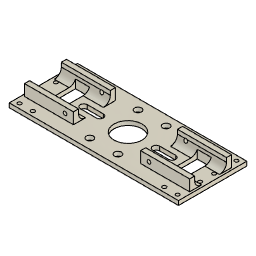
电路板支撑架 v2 (Autodesk Fusion 360 design; units mm, degrees)
Autodesk Fusion 360 part; units mm, degrees
sketch "草图1" plane through (0, 0, 0) normal (0, 0, 1) x (1, 0, 0)
  line L0 (-76.346, 23.9106) -> (50.654, 23.9106)
  line L1 (50.654, 23.9106) -> (50.654, -24.8894)
  line L2 (50.654, -24.8894) -> (-76.346, -24.8894)
  line L3 (-76.346, -24.8894) -> (-76.346, 23.9106)
  dimension "d1" = 127
  dimension "d2" = 48.8
  constraint horizontal L0
  constraint vertical L1
  constraint horizontal L2
  constraint vertical L3
  measures "d1" distance of L0.start L0.end
  measures "d2" distance of L0.start L2.end
extrude "拉伸1" add sketch "草图1" along normal blind 3
sketch "草图2" plane through (0, 0, 3) normal (0, 0, 1) x (-1, 0, 0)
  line L0 (76.346, 24.8894) -> (-50.654, 24.8894)
  line L1 (-50.654, 24.8894) -> (-50.654, -23.9106)
  line L2 (-50.654, -23.9106) -> (76.346, -23.9106)
  line L3 (76.346, -23.9106) -> (76.346, 24.8894)
  line L4 (12.846, -23.9106) -> (12.846, 24.8894) construction
  line L5 (76.346, 0.4894) -> (12.846, 0.4894) construction
  line L6 (12.846, 0.4894) -> (12.846, -12.4106)
  line L7 (-50.654, -10.9106) -> (76.346, -10.9106)
  line L8 (76.346, -10.9106) -> (76.346, -13.9106)
  line L9 (76.346, -13.9106) -> (-50.654, -13.9106)
  line L10 (-50.654, -13.9106) -> (-50.654, -10.9106)
  line L11 (-50.654, -10.9106) -> (76.346, -13.9106) construction
  line L12 (76.346, -10.9106) -> (-50.654, -13.9106) construction
  line L13 (12.846, 0.4894) -> (12.846, 13.3894)
  line L14 (-50.654, 14.8894) -> (76.346, 14.8894)
  line L15 (76.346, 14.8894) -> (76.346, 11.8894)
  line L16 (76.346, 11.8894) -> (-50.654, 11.8894)
  line L17 (-50.654, 11.8894) -> (-50.654, 14.8894)
  line L18 (-50.654, 14.8894) -> (76.346, 11.8894) construction
  line L19 (76.346, 14.8894) -> (-50.654, 11.8894) construction
  point P0 (12.846, -12.4106)
  point P1 (12.846, 13.3894)
  dimension "d5" = 12.9
  dimension "d6" = 3
  dimension "d7" = 3
  constraint midpoint L2 L4.start
  constraint midpoint L0 L4.end
  constraint midpoint L3 L5.start
  constraint midpoint L4 L5.end
  constraint perpendicular L5 L6
  constraint horizontal L7
  constraint perpendicular L7 L8
  constraint parallel L7 L9
  constraint parallel L8 L10
  constraint coincident L11 P0
  constraint coincident L12 P0
  constraint coincident P0 L6.end
  constraint symmetric L6.start L5 L13.start
  constraint symmetric L5 P0 P1
  constraint horizontal L14
  constraint perpendicular L14 L15
  constraint parallel L14 L16
  constraint parallel L15 L17
  constraint coincident L18 P1
  constraint coincident L19 P1
  constraint coincident P1 L13.end
  measures "d5" distance of L5.end P0
  measures "d6" distance of L7.end L8.end
  measures "d7" distance of L14.end L15.end
extrude "拉伸2" add sketch "草图2" along normal blind 8 contours L1 L3 L14 L15 L16 L17 | L1 L3 L7 L8 L9 L10
sketch "草图3" plane through (0, -14.8894, 0) normal (0, -1, 0) x (1, 0, 0)
  line L0 (-76.346, 3) -> (50.654, 3)
  line L1 (50.654, 3) -> (50.654, 11)
  line L2 (50.654, 11) -> (-76.346, 11)
  line L3 (-76.346, 11) -> (-76.346, 3)
  line L4 (-12.846, 11) -> (-12.846, 7)
  line L5 (-12.846, 7) -> (17.154, 7) construction
  circle A0 centre (17.154, 7) radius 1.3
  circle A1 centre (-42.846, 7) radius 1.3
  dimension "d13" = 4
  dimension "d14" = 30
  dimension "d15" = 2.6
  constraint midpoint L2 L4.start
  constraint perpendicular L2 L4
  constraint perpendicular L4 L5
  constraint coincident L5.end A0.centre
  constraint symmetric L4 A0 A1
  measures "d13" distance of L4.start L4.end
  measures "d14" distance of L4.end L5.end
  measures "d15" diameter of A0
extrude "拉伸3" cut sketch "草图3" against normal blind 28.8 contours A0 | A1
sketch "草图4" plane through (0, 13.9106, 0) normal (0, 1, 0) x (-1, 0, 0)
  circle A0 centre (-17.154, 7) radius 1.3
  circle A1 centre (42.846, 7) radius 1.3
  line L0 (-50.654, 3) -> (76.346, 3)
  line L1 (76.346, 3) -> (76.346, 11)
  line L2 (76.346, 11) -> (-50.654, 11)
  line L3 (-50.654, 11) -> (-50.654, 3)
  line L4 (12.846, 3) -> (12.846, 26.5) construction
  circle A2 centre (12.846, 26.5) radius 21
  dimension "d20" = 23.5
  dimension "d21" = 42
  constraint midpoint L0 L4.start
  constraint perpendicular L2 L4
  constraint coincident L4.end A2.centre
  measures "d20" distance of L4.start L4.end
  measures "d21" diameter of A2
sketch "草图5" plane through (0, 0, 0) normal (0, 0, -1) x (1, 0, 0)
  line L0 (50.654, 24.8894) -> (-76.346, 24.8894)
  line L1 (-76.346, 24.8894) -> (-76.346, -23.9106)
  line L2 (-76.346, -23.9106) -> (50.654, -23.9106)
  line L3 (50.654, -23.9106) -> (50.654, 24.8894)
  line L4 (-12.846, -23.9106) -> (-12.846, -3)
  line L5 (50.654, 0.4894) -> (30.654, 0.4894) construction
  line L6 (25.654, 11.4894) -> (35.654, 11.4894)
  line L7 (35.654, 11.4894) -> (35.654, -10.5106)
  line L8 (35.654, -10.5106) -> (25.654, -10.5106)
  line L9 (25.654, -10.5106) -> (25.654, 11.4894)
  line L10 (25.654, 11.4894) -> (35.654, -10.5106) construction
  line L11 (35.654, 11.4894) -> (25.654, -10.5106) construction
  line L12 (-51.346, -10.5106) -> (-51.346, 11.4894)
  line L13 (-61.346, -10.5106) -> (-51.346, -10.5106)
  line L14 (-61.346, 11.4894) -> (-61.346, -10.5106)
  line L15 (-51.346, 11.4894) -> (-61.346, 11.4894)
  circle A0 centre (-12.846, 0.4894) radius 10
  line L16 (30.654, 0.4894) -> (-51.346, 0.4894)
  line L17 (-12.846, -3) -> (-12.846, 0.4894)
  line L18 (-76.346, 24.8894) -> (-71.846, 24.8894)
  line L19 (-71.846, 24.8894) -> (-71.846, -23.9106)
  line L20 (-71.846, -23.9106) -> (-76.346, -23.9106)
  line L21 (-76.346, -23.9106) -> (-76.346, 24.8894)
  line L22 (46.154, 24.8894) -> (46.154, -23.9106)
  line L23 (50.654, -23.9106) -> (50.654, 24.8894)
  line L24 (50.654, 24.8894) -> (46.154, 24.8894)
  line L25 (46.154, -23.9106) -> (50.654, -23.9106)
  point P0 (30.654, 0.4894)
  dimension "d24" = 20
  dimension "d25" = 10
  dimension "d26" = 22
  dimension "d29" = 20
  dimension "d54" = 4.5
  dimension "d55" = 48.8
  constraint midpoint L2 L4.start
  constraint perpendicular L2 L4
  constraint midpoint L3 L5.start
  constraint perpendicular L3 L5
  constraint horizontal L6
  constraint perpendicular L6 L7
  constraint parallel L6 L8
  constraint parallel L7 L9
  constraint coincident L10 P0
  constraint coincident L11 P0
  constraint coincident P0 L5.end
  constraint symmetric L4 L6.start L12.end
  constraint symmetric L4 L6.end L14.start
  constraint symmetric L4 L7.end L13.start
  constraint symmetric L4 L8.end L12.start
  constraint midpoint L12 L16.end
  constraint coincident A0.centre L16
  constraint coincident L16 A0.centre
  constraint perpendicular L16 L17
  constraint coincident A0.centre L17.end
  constraint horizontal L18
  constraint vertical L19
  constraint horizontal L20
  constraint vertical L21
  constraint coincident L0.end L1.start
  constraint symmetric L17 L0.end L0.start
  constraint symmetric L17 L18.end L22.start
  constraint symmetric L17 L19.end L22.end
  constraint symmetric L17 L1.end L2.end
  measures "d24" distance of L5.start P0
  measures "d25" distance of L7.end L8.end
  measures "d26" distance of L6.end L7.end
  measures "d29" diameter of A0
  measures "d54" distance of L0.end L18.end
  measures "d55" distance of L0.end L1.end
extrude "拉伸5" cut sketch "草图5" against normal blind 3 contours L6 L7 L8 L9 | L12 L13 L14 L15
extrude "拉伸6" cut sketch "草图5" against normal blind 3 contours L4 A0 L16 L17 | L4 A0 L16 L17 | A0 L16
fillet "圆角2" radius 5 2 edges at (-12.846, 10.9106, 3) (-12.846, -11.8894, 3)
sketch "草图6" plane through (0, -14.8894, 0) normal (0, -1, 0) x (1, 0, 0)
  circle A0 centre (17.154, 7) radius 1.3
  circle A1 centre (-42.846, 7) radius 1.3
  line L0 (-76.346, 3) -> (50.654, 3)
  line L1 (50.654, 3) -> (50.654, 11)
  line L2 (50.654, 11) -> (-76.346, 11)
  line L3 (-76.346, 11) -> (-76.346, 3)
  line L4 (17.154, 7) -> (-12.846, 7)
  line L5 (11.154, 11) -> (-36.846, 11)
  line L6 (-36.846, 11) -> (-36.846, 3)
  line L7 (-36.846, 3) -> (11.154, 3)
  line L8 (11.154, 3) -> (11.154, 11)
  line L9 (11.154, 11) -> (-36.846, 3) construction
  line L10 (-36.846, 11) -> (11.154, 3) construction
  point P0 (-12.846, 7)
  dimension "d34" = 30
  dimension "d35" = 48
  constraint coincident A0.centre L4.start
  constraint parallel L0 L4
  constraint horizontal L5
  constraint perpendicular L5 L6
  constraint parallel L5 L7
  constraint parallel L6 L8
  constraint coincident L9 P0
  constraint coincident L10 P0
  constraint coincident L2 L5.start
  constraint coincident P0 L4.end
  measures "d34" distance of A0.centre P0
  measures "d35" distance of L6.end L7.end
extrude "拉伸7" cut sketch "草图6" against normal blind 28.8 contours L0 L2 L5 L6 L7 L8
sketch "草图7" plane through (0, 0, 0) normal (0, 0, -1) x (1, 0, 0)
  circle A0 centre (-12.846, 0.4894) radius 10
  line L0 (-61.346, -10.5106) -> (-61.346, 11.4894)
  line L1 (-61.346, 11.4894) -> (-51.346, 11.4894)
  line L2 (-51.346, 11.4894) -> (-51.346, -10.5106)
  line L3 (-51.346, -10.5106) -> (-61.346, -10.5106)
  line L4 (35.654, 11.4894) -> (35.654, -10.5106)
  line L5 (35.654, -10.5106) -> (25.654, -10.5106)
  line L6 (25.654, -10.5106) -> (25.654, 11.4894)
  line L7 (25.654, 11.4894) -> (35.654, 11.4894)
  line L8 (50.654, 24.8894) -> (-76.346, 24.8894)
  line L9 (-76.346, 24.8894) -> (-76.346, -23.9106)
  line L10 (-76.346, -23.9106) -> (50.654, -23.9106)
  line L11 (50.654, -23.9106) -> (50.654, 24.8894)
  line L12 (34.154, -20.5106) -> (-59.846, -20.5106) construction
  line L13 (-59.846, -20.5106) -> (-59.846, 21.4894) construction
  line L14 (-59.846, 21.4894) -> (34.154, 21.4894) construction
  line L15 (34.154, 21.4894) -> (34.154, -20.5106) construction
  line L16 (34.154, -20.5106) -> (-59.846, 21.4894) construction
  line L17 (-59.846, -20.5106) -> (34.154, 21.4894) construction
  circle A1 centre (-59.846, 21.4894) radius 1.4
  circle A2 centre (34.154, 21.4894) radius 1.4
  circle A3 centre (34.154, -20.5106) radius 1.4
  circle A4 centre (-59.846, -20.5106) radius 1.4
  point P0 (-12.846, 0.4894)
  dimension "d38" = 94
  dimension "d39" = 42
  dimension "d40" = 2.8
  dimension "d41" = 2.8
  dimension "d42" = 2.8
  dimension "d43" = 2.8
  constraint horizontal L12
  constraint perpendicular L12 L13
  constraint parallel L12 L14
  constraint parallel L13 L15
  constraint coincident L16 P0
  constraint coincident L17 P0
  constraint coincident P0 A0.centre
  constraint coincident L13.end L14.start
  constraint coincident L14.end L15.start
  constraint coincident L12.start L15.end
  constraint coincident L12.end L13.start
  measures "d38" distance of L13.end L14.end
  measures "d39" distance of L12.end L13.end
  measures "d40" diameter of A1
  measures "d41" diameter of A2
  measures "d42" diameter of A3
  measures "d43" diameter of A4
extrude "拉伸8" cut sketch "草图7" against normal blind 3 contours A1 | A2 | A3 | A4
sketch "草图8" plane through (0, 0, 3) normal (0, 0, 1) x (-1, 0, 0)
  circle A0 centre (59.846, -20.5106) radius 1.4
  circle A1 centre (-34.154, 21.4894) radius 1.4
  circle A2 centre (59.846, 21.4894) radius 1.4
  circle A3 centre (-34.154, -20.5106) radius 1.4
  circle A4 centre (12.846, 0.4894) radius 10
  line L0 (-50.654, 14.8894) -> (-11.154, 14.8894)
  line L1 (-11.154, 14.8894) -> (-11.154, 6.8894)
  line L2 (-11.154, 6.8894) -> (-25.654, 6.8894)
  line L3 (-25.654, 6.8894) -> (-25.654, -5.9106)
  line L4 (-25.654, -5.9106) -> (-11.154, -5.9106)
  line L5 (-11.154, -5.9106) -> (-11.154, -13.9106)
  line L6 (-11.154, -13.9106) -> (-50.654, -13.9106)
  line L7 (-50.654, -13.9106) -> (-50.654, -23.9106)
  line L8 (-50.654, -23.9106) -> (76.346, -23.9106)
  line L9 (76.346, -23.9106) -> (76.346, -13.9106)
  line L10 (76.346, -13.9106) -> (36.846, -13.9106)
  line L11 (36.846, -13.9106) -> (36.846, -5.9106)
  line L12 (36.846, -5.9106) -> (51.346, -5.9106)
  line L13 (51.346, -5.9106) -> (51.346, 6.8894)
  line L14 (51.346, 6.8894) -> (36.846, 6.8894)
  line L15 (36.846, 6.8894) -> (36.846, 14.8894)
  line L16 (36.846, 14.8894) -> (76.346, 14.8894)
  line L17 (76.346, 14.8894) -> (76.346, 24.8894)
  line L18 (76.346, 24.8894) -> (-50.654, 24.8894)
  line L19 (-50.654, 24.8894) -> (-50.654, 14.8894)
  line L20 (-33.654, 21.4894) -> (59.346, 21.4894)
  line L21 (59.346, 21.4894) -> (59.346, -20.5106)
  line L22 (59.346, -20.5106) -> (-33.654, -20.5106)
  line L23 (-33.654, -20.5106) -> (-33.654, 21.4894)
  line L24 (-33.654, 21.4894) -> (59.346, -20.5106) construction
  line L25 (59.346, 21.4894) -> (-33.654, -20.5106) construction
  point P0 (12.846, 0.4894)
  dimension "d46" = 93
  dimension "d47" = 42
  constraint horizontal L20
  constraint perpendicular L20 L21
  constraint parallel L20 L22
  constraint parallel L21 L23
  constraint coincident L24 P0
  constraint coincident L25 P0
  constraint coincident P0 A4.centre
  measures "d46" distance of L21.end L22.end
  measures "d47" distance of L20.end L21.end
sketch "草图9" plane through (0, 0, 3) normal (0, 0, 1) x (-1, 0, 0)
  circle A0 centre (59.846, -20.5106) radius 1.4
  circle A1 centre (-34.154, 21.4894) radius 1.4
  circle A2 centre (59.846, 21.4894) radius 1.4
  circle A3 centre (-34.154, -20.5106) radius 1.4
  circle A4 centre (12.846, 0.4894) radius 10
  line L0 (-50.654, 14.8894) -> (-11.154, 14.8894)
  line L1 (-11.154, 14.8894) -> (-11.154, 6.8894)
  line L2 (-11.154, 6.8894) -> (-25.654, 6.8894)
  line L3 (-25.654, 6.8894) -> (-25.654, -5.9106)
  line L4 (-25.654, -5.9106) -> (-11.154, -5.9106)
  line L5 (-11.154, -5.9106) -> (-11.154, -13.9106)
  line L6 (-11.154, -13.9106) -> (-50.654, -13.9106)
  line L7 (-50.654, -13.9106) -> (-50.654, -23.9106)
  line L8 (-50.654, -23.9106) -> (76.346, -23.9106)
  line L9 (76.346, -23.9106) -> (76.346, -13.9106)
  line L10 (76.346, -13.9106) -> (36.846, -13.9106)
  line L11 (36.846, -13.9106) -> (36.846, -5.9106)
  line L12 (36.846, -5.9106) -> (51.346, -5.9106)
  line L13 (51.346, -5.9106) -> (51.346, 6.8894)
  line L14 (51.346, 6.8894) -> (36.846, 6.8894)
  line L15 (36.846, 6.8894) -> (36.846, 14.8894)
  line L16 (36.846, 14.8894) -> (76.346, 14.8894)
  line L17 (76.346, 14.8894) -> (76.346, 24.8894)
  line L18 (76.346, 24.8894) -> (-50.654, 24.8894)
  line L19 (-50.654, 24.8894) -> (-50.654, 14.8894)
  circle A5 centre (12.846, 0.4894) radius 20 construction
  circle A6 centre (32.8457, 0.5905) radius 2.5
  circle A7 centre (22.7583, 17.8603) radius 2.5
  circle A8 centre (2.7586, 17.7592) radius 2.5
  circle A9 centre (-7.1538, 0.3884) radius 2.5
  circle A10 centre (2.9336, -16.8814) radius 2.5
  circle A11 centre (22.9334, -16.7803) radius 2.5
  line L20 (-7.1538, 2.8884) -> (-18.6538, 2.8884)
  arc A12 (-18.6538, 2.8884) -> (-18.6538, -2.1116) centre (-18.6538, 0.3884) ccw
  line L21 (-18.6538, -2.1116) -> (-7.1538, -2.1116)
  arc A13 (-7.1538, -2.1116) -> (-7.1538, 2.8884) centre (-7.1538, 0.3884) ccw
  line L22 (-7.1538, 0.3884) -> (-18.6538, 0.3884) construction
  line L23 (32.8457, -1.9095) -> (44.3457, -1.9095)
  arc A14 (44.3457, -1.9095) -> (44.3457, 3.0905) centre (44.3457, 0.5905) ccw
  line L24 (44.3457, 3.0905) -> (32.8457, 3.0905)
  arc A15 (32.8457, 3.0905) -> (32.8457, -1.9095) centre (32.8457, 0.5905) ccw
  line L25 (32.8457, 0.5905) -> (44.3457, 0.5905) construction
  dimension "d48" = 40
  dimension "d49" = 5
  dimension "d51" = 360
  dimension "d62" = 11.5
  constraint concentric A4 A5
  constraint coincident A5 A6.centre
  constraint tangent L20 A12
  constraint tangent A12 L21
  constraint parallel L20 L21
  constraint tangent L21 A13
  constraint tangent L20 A13
  constraint horizontal L22
  constraint coincident A9.centre A13.centre
  constraint tangent L23 A14
  constraint tangent A14 L24
  constraint parallel L23 L24
  constraint tangent L24 A15
  constraint tangent L23 A15
  constraint horizontal L25
  constraint coincident A6.centre A15.centre
  measures "d48" diameter of A5
  measures "d49" diameter of A6
  measures "d62" distance of A9.centre A12.centre
extrude "拉伸9" cut sketch "草图9" against normal blind 3 contours A6 A15 | A7 | A8 | A9 A13 | A10 | A11
extrude "拉伸10" cut sketch "草图5" against normal blind 11 contours L0 L2 L3 L22 L23 L24 L25 | L0 L1 L2 L18 L19 L20 L21
extrude "拉伸11" add 2 faces at (36.9207, -14.8894, 7) (-62.6126, -14.8894, 7) along direction (0, -1, 0) blind 0.6
extrude "拉伸12" add 2 faces at (-62.6126, 13.9106, 7) (36.9207, 13.9106, 7) along direction (0, 1, 0) blind 0.6
extrude "拉伸13" cut sketch "草图9" against normal blind 3 contours A6 L23 A14 L24 | A9 L20 A12 L21
sketch "草图10" plane through (-71.846, 0, 0) normal (-1, 0, 0) x (0, -1, 0)
  line L0 (11.8894, 11) -> (11.8894, 8)
  arc A0 (6.8894, 3) -> (11.8894, 8) centre (6.8894, 8) ccw
  line L1 (6.8894, 3) -> (-5.9106, 3)
  arc A1 (-10.9106, 8) -> (-5.9106, 3) centre (-5.9106, 8) ccw
  line L2 (-10.9106, 8) -> (-10.9106, 11)
  line L3 (-10.9106, 11) -> (-14.5106, 11)
  line L4 (-14.5106, 11) -> (-14.5106, 3)
  line L5 (-14.5106, 3) -> (-23.9106, 3)
  line L6 (-23.9106, 3) -> (-23.9106, 0)
  line L7 (-23.9106, 0) -> (24.8894, 0)
  line L8 (24.8894, 0) -> (24.8894, 3)
  line L9 (24.8894, 3) -> (15.4894, 3)
  line L10 (15.4894, 3) -> (15.4894, 11)
  line L11 (15.4894, 11) -> (11.8894, 11)
sketch "草图11" plane through (-71.846, 0, 0) normal (-1, 0, 0) x (0, -1, 0)
  line L0 (11.8894, 11) -> (11.8894, 8)
  arc A0 (6.8894, 3) -> (11.8894, 8) centre (6.8894, 8) ccw
  line L1 (6.8894, 3) -> (-5.9106, 3)
  arc A1 (-10.9106, 8) -> (-5.9106, 3) centre (-5.9106, 8) ccw
  line L2 (-10.9106, 8) -> (-10.9106, 11)
  line L3 (-10.9106, 11) -> (-14.5106, 11)
  line L4 (-14.5106, 11) -> (-14.5106, 3)
  line L5 (-14.5106, 3) -> (-23.9106, 3)
  line L6 (-23.9106, 3) -> (-23.9106, 0)
  line L7 (-23.9106, 0) -> (24.8894, 0)
  line L8 (24.8894, 0) -> (24.8894, 3)
  line L9 (24.8894, 3) -> (15.4894, 3)
  line L10 (15.4894, 3) -> (15.4894, 11)
  line L11 (15.4894, 11) -> (11.8894, 11)
  line L12 (-23.9106, 3) -> (24.8894, 3)
  line L13 (24.8894, 3) -> (24.8894, 0)
  line L14 (24.8894, 0) -> (-23.9106, 0)
  line L15 (-23.9106, 0) -> (-23.9106, 3)
  constraint horizontal L12
  constraint vertical L13
  constraint horizontal L14
  constraint vertical L15
  constraint coincident L7.end L8.start
  constraint coincident L5.end L6.start
extrude "拉伸14" add sketch "草图11" along normal blind 1.5 contours L1 L5 L6 L7 L8 L9 L12 L13 L14 L15
sketch "草图12" plane through (46.154, 0, 0) normal (1, 0, 0) x (0, 1, 0)
  line L0 (-11.8894, 8) -> (-11.8894, 11)
  line L1 (-11.8894, 11) -> (-15.4894, 11)
  line L2 (-15.4894, 11) -> (-15.4894, 3)
  line L3 (-15.4894, 3) -> (-24.8894, 3)
  line L4 (-24.8894, 3) -> (-24.8894, 0)
  line L5 (-24.8894, 0) -> (23.9106, 0)
  line L6 (23.9106, 0) -> (23.9106, 3)
  line L7 (23.9106, 3) -> (14.5106, 3)
  line L8 (14.5106, 3) -> (14.5106, 11)
  line L9 (14.5106, 11) -> (10.9106, 11)
  line L10 (10.9106, 11) -> (10.9106, 8)
  arc A0 (5.9106, 3) -> (10.9106, 8) centre (5.9106, 8) ccw
  line L11 (5.9106, 3) -> (-6.8894, 3)
  arc A1 (-11.8894, 8) -> (-6.8894, 3) centre (-6.8894, 8) ccw
  line L12 (23.9106, 0) -> (-24.8894, 0)
  line L13 (-24.8894, 0) -> (-24.8894, 3)
  line L14 (-24.8894, 3) -> (23.9106, 3)
  line L15 (23.9106, 3) -> (23.9106, 0)
  constraint horizontal L12
  constraint vertical L13
  constraint horizontal L14
  constraint vertical L15
  constraint coincident L3.end L4.start
  constraint coincident L5.end L6.start
extrude "拉伸15" add sketch "草图12" along normal blind 1.5 contours L3 L4 L5 L6 L7 L11 L12 L13 L14 L15
sketch "草图13" plane through (0, 0, 0) normal (0, 0, -1) x (1, 0, 0)
  line L0 (-44.3457, 3.0905) -> (-32.8457, 3.0905)
  arc A0 (-32.8457, -1.9095) -> (-32.8457, 3.0905) centre (-32.8457, 0.5905) ccw
  line L1 (-32.8457, -1.9095) -> (-44.3457, -1.9095)
  arc A1 (-44.3457, 3.0905) -> (-44.3457, -1.9095) centre (-44.3457, 0.5905) ccw
  line L2 (18.6538, -2.1116) -> (7.1538, -2.1116)
  arc A2 (7.1538, 2.8884) -> (7.1538, -2.1116) centre (7.1538, 0.3884) ccw
  line L3 (7.1538, 2.8884) -> (18.6538, 2.8884)
  arc A3 (18.6538, -2.1116) -> (18.6538, 2.8884) centre (18.6538, 0.3884) ccw
  line L4 (47.654, 24.8894) -> (-73.346, 24.8894)
  line L5 (-73.346, 24.8894) -> (-73.346, -23.9106)
  line L6 (-73.346, -23.9106) -> (47.654, -23.9106)
  line L7 (47.654, -23.9106) -> (47.654, 24.8894)
  circle A4 centre (-2.9336, -16.8814) radius 2.5
  circle A5 centre (-2.7586, 17.7592) radius 2.5
  circle A6 centre (-22.9334, -16.7803) radius 2.5
  circle A7 centre (-22.7583, 17.8603) radius 2.5
  circle A8 centre (-59.846, -20.5106) radius 1.4
  circle A9 centre (34.154, 21.4894) radius 1.4
  circle A10 centre (-59.846, 21.4894) radius 1.4
  circle A11 centre (34.154, -20.5106) radius 1.4
  circle A12 centre (-12.846, 0.4894) radius 10
  line L8 (-61.346, -10.5106) -> (-61.346, 11.4894)
  line L9 (-61.346, 11.4894) -> (-51.346, 11.4894)
  line L10 (-51.346, 11.4894) -> (-51.346, -10.5106)
  line L11 (-51.346, -10.5106) -> (-61.346, -10.5106)
  line L12 (35.654, 11.4894) -> (35.654, -10.5106)
  line L13 (35.654, -10.5106) -> (25.654, -10.5106)
  line L14 (25.654, -10.5106) -> (25.654, 11.4894)
  line L15 (25.654, 11.4894) -> (35.654, 11.4894)
  line L16 (-73.346, 0.4894) -> (-69.346, 0.4894)
  line L17 (-69.346, 0.4894) -> (-69.346, 5.4894)
  circle A13 centre (-69.346, 5.4894) radius 1.3
  line L18 (-59.846, 21.4894) -> (-69.346, 21.4894)
  circle A14 centre (-69.346, 21.4894) radius 1.3
  circle A15 centre (-69.346, -20.5106) radius 1.3
  circle A16 centre (-69.346, -4.5106) radius 1.3
  line L19 (-12.846, 0.4894) -> (-12.846, 6)
  circle A17 centre (43.654, 21.4894) radius 1.3
  circle A18 centre (43.654, 5.4894) radius 1.3
  circle A19 centre (43.654, -4.5106) radius 1.3
  circle A20 centre (43.654, -20.5106) radius 1.3
  dimension "d71" = 4
  dimension "d72" = 5
  dimension "d73" = 2.6
  dimension "d74" = 2.6
  constraint midpoint L5 L16.start
  constraint perpendicular L5 L16
  constraint perpendicular L16 L17
  constraint coincident L17.end A13.centre
  constraint coincident A10.centre L18.start
  constraint perpendicular L17 L18
  constraint coincident L18.end A14.centre
  constraint symmetric L16 A13 A16
  constraint symmetric L16 A14 A15
  constraint coincident A12.centre L19.start
  constraint vertical L19
  constraint symmetric A13 L19 A18
  constraint symmetric A14 L19 A17
  constraint symmetric A15 L19 A20
  constraint symmetric A16 L19 A19
  measures "d71" distance of L16.start L16.end
  measures "d72" distance of L16.end L17.end
  measures "d73" diameter of A13
  measures "d74" diameter of A14
extrude "拉伸16" cut sketch "草图13" against normal blind 3 contours A13 | A14 | A15 | A16 | A17 | A18 | A19 | A20
equation "d34 = ( 60 / 2 ) * 1 mm"
